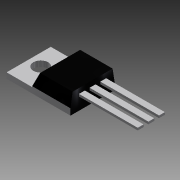
# Autodesk Inventor part: MOSFET
Saved by Autodesk Inventor 2014 (Build 180170000, 170)
## iProperties
Created: 2015-04-18
Part Number: MOSFET
Material: Generic
Document SubType Name: Modeling
Designer: Owner
Density: 1 g/cm^3
Appearance: Default
Author: Owner
Autodesk Inventor part; units mm, degrees
ref_plane "YZ Plane" through (0, 0, 0) normal (1, 0, 0) x (0, 1, 0)
ref_plane "XZ Plane" through (0, 0, 0) normal (0, 1, 0) x (-1, 0, 0)
ref_plane "XY Plane" through (0, 0, 0) normal (0, 0, 1) x (1, 0, 0)
sketch "Sketch1" plane through (0, 0, 0) normal (0, 1, 0) x (-1, 0, 0)
  line L0 (-7.0894, 4.7564) -> (8.1506, 4.7564)
  line L1 (8.1506, 4.7564) -> (8.1506, -5.7836)
  line L2 (8.1506, -5.7836) -> (-7.0894, -5.7836)
  line L3 (-7.0894, -5.7836) -> (-7.0894, 4.7564)
  circle A0 centre (5.2806, -0.5136) radius 1.77
  point P0 (0, 0)
  dimension "d0" = 10.54
  dimension "d1" = 15.24
  dimension "d2" = 3.54
  dimension "d3" = 2.87
  dimension "d4" = 5.27
  constraints: 8 end point, 2 parallel, 1 centre point, 1 horizontal, 1 perpendicular
  measures "d0" distance of L0.end L1.end
  measures "d1" distance of L0.start L0.end
  measures "d2" diameter of A0
  measures "d3" distance from line of L1 A0.centre
  measures "d4" distance from line of A0.centre L0
extrude "Extrusion1" add sketch "Sketch1" along normal blind 1.32
sketch "Sketch2" plane through (0, 1.32, 0) normal (0, 1, 0) x (1, 0, 0)
  line L0 (7.0894, 5.7836) -> (-8.1506, 5.7836) projected
  line L1 (-2.0506, 5.7836) -> (7.0894, 5.7836)
  line L2 (7.0894, 5.7836) -> (7.0894, -4.7564)
  line L3 (7.0894, -4.7564) -> (-2.0506, -4.7564)
  line L4 (-2.0506, -4.7564) -> (-2.0506, 5.7836)
  point P0 (0, 0)
  dimension "d7" = 9.14
  constraints: 8 end point, 2 parallel, 1 horizontal, 1 perpendicular, 1 point on line
  measures "d7" distance of L2.end L3.end
extrude "Extrusion2" add sketch "Sketch2" along normal blind 3.37
chamfer "Chamfer1" distance 1.4 distance2 3.175 1 edges at (-2.0506, 4.69, -0.5136) measured on face at (0.996, 4.69, -2.2703)
chamfer "Chamfer2" distance 0.5 distance2 3.175 1 edges at (3.2194, 4.69, -5.7836) measured on face at (1.9294, 4.69, -2.2703)
chamfer "Chamfer3" distance 0.5 distance2 3.175 1 edges at (3.2194, 4.69, 4.7564) measured on face at (1.9294, 4.69, -1.9369)
sketch "Sketch4" plane through (7.0894, 0, 4.7564) normal (1, 0, 0) x (0, 0, -1)
  line L0 (0, 0) -> (0, 1.515) projected
  line L1 (10.54, 0) -> (0, 0) projected
  line L2 (2.03, 3.47) -> (8.51, 3.47)
  line L3 (8.51, 3.47) -> (8.51, 2.92)
  line L4 (8.51, 2.92) -> (2.03, 2.92)
  line L5 (2.03, 2.92) -> (2.03, 3.47)
  line L6 (3.43, 3.47) -> (3.43, 2.92)
  line L7 (4.57, 3.47) -> (4.57, 2.92)
  line L8 (5.97, 3.47) -> (5.97, 2.92)
  line L9 (7.11, 3.47) -> (7.11, 2.92)
  point P0 (4.7564, 0)
  dimension "d19" = 0.55
  dimension "d20" = 2.92
  dimension "d21" = 6.48
  dimension "d22" = 1.4
  dimension "d23" = 1.4
  dimension "d24" = 1.4
  dimension "d25" = 2.54
  dimension "d26" = 4.57
  constraints: 16 end point, 8 point on line, 5 perpendicular, 2 parallel, 1 horizontal
  measures "d19" distance of L2.end L3.end
  measures "d20" distance between parallel lines of L1 L4
  measures "d21" distance of L2.start L2.end
  measures "d22" distance between parallel lines of L3 L9
  measures "d23" distance between parallel lines of L7 L8
  measures "d24" distance between parallel lines of L5 L6
  measures "d25" distance between parallel lines of L8 L6
  measures "d26" distance between parallel lines of L0 L7
extrude "Extrusion3" add sketch "Sketch4" along normal blind 14 contours L2 L6 L4 L5 | L2 L8 L4 L7 | L2 L3 L4 L9
body "Solid1"
